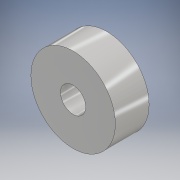
# Autodesk Inventor part: BEARING
Saved by Autodesk Inventor 2017 (Build 210142000, 142)
## iProperties
Created: 2017-09-24
Part Number: BEARING
Material: Generic
Document SubType Name: Modeling
Designer: Alexander Miller
Density: 1 g/cm^3
Appearance: Aluminum - Dark
bearing_A: 10,000 mm
bearing_B: 3,000 mm
bearing_C: 4,000 mm
Author: Alexander Miller
Autodesk Inventor part; units mm, degrees
ref_plane "YZ Plane" through (0, 0, 0) normal (1, 0, 0) x (0, 1, 0)
ref_plane "XZ Plane" through (0, 0, 0) normal (0, 1, 0) x (-1, 0, 0)
ref_plane "XY Plane" through (0, 0, 0) normal (0, 0, 1) x (1, 0, 0)
sketch "Sketch1" plane through (0, 0, 0) normal (0, 1, 0) x (-1, 0, 0)
  circle A0 centre (0, 0) radius 5
  circle A1 centre (0, 0) radius 1.5
  dimension "d0" = 3
  dimension "d1" = 10
  constraints: 2 centre point, 1 coincident, 1 concentric
  measures "d0" diameter of A1
  measures "d1" diameter of A0
extrude "Extrusion1" add sketch "Sketch1" along normal blind 4
equation "\"d0\" = bearing_B"
equation "\"d1\" = bearing_A"
equation "\"d2\" = bearing_C"
equation "\"bearing_A\" = 10"
equation "\"bearing_B\" = 3"
equation "\"bearing_C\" = 4"
body "Solid1"
